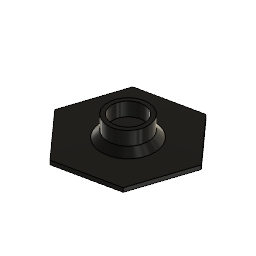
twisted top (Autodesk Fusion 360 design; units mm, degrees)
part number: 2026-05-21-00-01-04-472
Autodesk Fusion 360 part; units mm, degrees
sketch "Sketch1" plane through (0, 0, 0) normal (0, 0, 1) x (1, 0, 0)
  line L0 (-25.748, 28.7303) -> (11.9841, 36.6874)
  line L1 (11.9841, 36.6874) -> (37.7548, 7.9326)
  line L2 (37.7548, 7.9326) -> (25.748, -28.7303)
  line L3 (25.748, -28.7303) -> (-11.9841, -36.6874)
  line L4 (-11.9841, -36.6874) -> (-37.7548, -7.9326)
  line L5 (-37.7548, -7.9326) -> (-25.748, 28.7303)
  line L6 (-25.748, 28.7303) -> (25.748, -28.7303) construction
  dimension "d1" = 38.562
  dimension "d2" = 38.562
  dimension "d3" = 38.613
  dimension "d4" = 38.613
  dimension "d5" = 38.579
  dimension "d6" = 38.579
  dimension "d7" = 66.85
  dimension "d8" = 66.82
  constraint parallel L0 L3
  constraint parallel L1 L4
  constraint midpoint origin L6
  measures "d1" distance of L0.start L0.end
  measures "d2" distance of L2.end L3.end
  measures "d3" distance of L0.end L1.end
  measures "d4" distance of L3.end L4.end
  measures "d5" distance of L1.end L2.end
  measures "d6" distance of L0.start L4.end
  measures "d7" distance of L0 L3
  measures "d8" distance of L1 L4
extrude "Extrude1" add sketch "Sketch1" along normal blind 2.5
sketch "Sketch2" plane through (0, 0, 2.5) normal (0, 0, 1) x (-1, 0, 0)
  line L0 (37.7548, 7.9326) -> (11.9841, 36.6874)
  line L1 (11.9841, 36.6874) -> (-25.748, 28.7303)
  line L2 (-25.748, 28.7303) -> (-37.7548, -7.9326)
  line L3 (-37.7548, -7.9326) -> (-11.9841, -36.6874)
  line L4 (-11.9841, -36.6874) -> (25.748, -28.7303)
  line L5 (25.748, -28.7303) -> (37.7548, 7.9326)
  circle A0 centre (0, 0) radius 16.5
  dimension "d11" = 33
  constraint coincident A0.centre origin
  measures "d11" diameter of A0
extrude "Extrude2" add sketch "Sketch2" along normal blind 4 draft -45 contours A0
sketch "Sketch3" plane through (0, 0, 6.5) normal (0, 0, 1) x (-1, 0, 0)
  circle A0 centre (0, 0) radius 12.5
  circle A1 centre (0, 0) radius 10
  circle A2 centre (0, 0) radius 12.5
  dimension "d14" = 20
  dimension "d15" = 25
  constraint coincident A0.centre A1.centre
  constraint concentric A1 A2
  measures "d14" diameter of A1
  measures "d15" diameter of A2
extrude "Extrude3" add sketch "Sketch3" along normal blind 8.5
